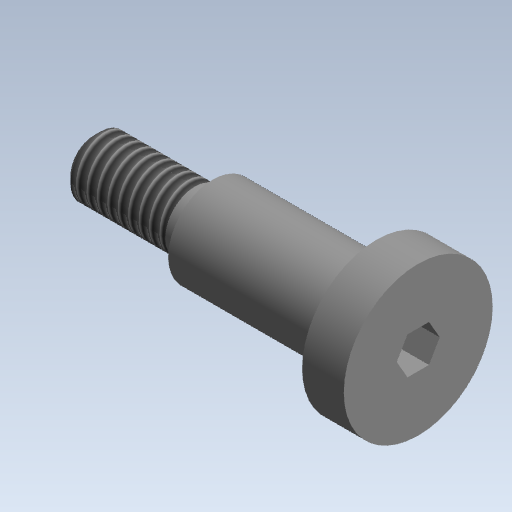
# Autodesk Inventor part: DBTS4-11-8
Saved by Autodesk Inventor 2020.4 (Build 244396000, 396)
## iProperties
Part Number: DBTS4-11-8
Material: 一般
Catalog Web Link: https://jp.misumi-ec.com/vona2/detail/110302679110/?HissuCode=DBTS4-11-8
Description: 既製品
Vendor: MISUMI
Document SubType Name: Modeling
Designer: partserver
Manufacturer: MISUMI
Mass: 0.615672 g
Surface Area: 5.71929 cm^2
Volume: 0.615672 cm^3
Density: 1 g/cm^3
Appearance: PSOLRGB-175-175-175
Category: PARTsolutions
Company: MISUMI
PSOL_IDENT_0: {$CADENAS_DATA\23d-libs\misumi\metric\27_screws_nuts\dbtb.prj},198 {VTYP=3D},{NB=DBTS4-11-8},{LINA=D
PSOL_IDENT_1: BTS4-11-8},{NN=DBTB, DBTM, DBTS},{DATE=03.06.2021 03:35:29},{GEOMDATE=06.03.2020 06:09:28},{VERSION=
PSOL_IDENT_2: },{LINEID=20},{WBVAR=MAT,ST,ALT1,L,F,ALT2,ALT3},{WBNUMERIC=L,F}  {NB=DBTS4-11-8},{LINA=DBTS4-11-8},{
PSOL_IDENT_3: KT=DUMMY},{PN=DBTS4-11-8},{TYPE=DBTS},{MAT=2},{ST=0},{ST0='0','-'},{M=4},{ALT1=},{L=11},{F=8},{FA=(3
PSOL_IDENT_4: :9/1)},{E=2.8},{D=6},{A=10},{B=2.5},{LL=1.2},{HH1=2.5},{P=0.7},{ALT2=},{GG=0.0},{FF=0.0},{LINC=[3:20
PSOL_IDENT_5: /1]},{ALT3=},{TOL=0/-0.2}
NB: DBTS4-11-8
NN: DBTB, DBTM, DBTS
NT: Stepped Bolts - Low Head Type
NBSYN: $PN.
LINA: DBTS4-11-8
CATALOG: Misumi
PN: DBTS4-11-8
MAT: 303 Stainless Steel
ST: -
M: 4
ALT1: w/o LTC (L Dimension Increment)
L: 11
F: 8
E: 2.8
D: 6
A: 10
B: 2.5
LL: 1.2
HH1: 2.5
ALT2: w/o PC (Relief on M)
ALT3: w/o DHC (Shaft Diameter Tolerance)
TOL: 0/-0.2
SUPPLIER: MISUMI
ARTICLENO: DBTS4-11-8
BOMINFO: DBTS4-11-8
CREATOR: CADENAS GmbH
Title: DBTS4-11-8
Author: Cadenas PARTsolutions
Comments: Stepped Bolts - Low Head Type
Autodesk Inventor part; units mm, degrees
ref_plane "YZ Plane" through (0, 0, 0) normal (1, 0, 0) x (0, 1, 0)
ref_plane "XZ Plane" through (0, 0, 0) normal (0, 1, 0) x (-1, 0, 0)
ref_plane "XY Plane" through (0, 0, 0) normal (0, 0, 1) x (1, 0, 0)
sketch "Sketch_1" plane through (0, 0, 0) normal (0, 0, 1) x (1, 0, 0)
  line L0 (11, 0) -> (-2.8, 0)
  line L1 (-2.8, 0) -> (-2.8, 5)
  line L2 (-2.8, 5) -> (0, 5)
  line L3 (0, 5) -> (0, 3)
  line L4 (0, 3) -> (11, 3)
  line L5 (11, 3) -> (11, 0)
  line L6 (11, 0) -> (-2.8, 0)
  constraints: 14 end point
revolve "Revolution1" add sketch "Sketch_1" angle 360 about axis through (11, 0, 0) along (1, 0, 0)
sketch "Sketch2" plane through (-2.8, 0, 0) normal (-1, 0, 0) x (0, 0, 1)
  point P0 (0, 0)
hole "Hole1" at (-2.8, 0, 0) direction (1, 0, 0) diameter 2.5 depth 2.5 tip angle 120
sketch "Sketch_3" plane through (-2.8, 0, 0) normal (1, 0, 0) x (0, 0, -1)
  line L0 (-1.25, -0.7217) -> (0, -1.4434)
  line L1 (0, -1.4434) -> (1.25, -0.7217)
  line L2 (1.25, -0.7217) -> (1.25, 0.7217)
  line L3 (1.25, 0.7217) -> (0, 1.4434)
  line L4 (0, 1.4434) -> (-1.25, 0.7217)
  line L5 (-1.25, 0.7217) -> (-1.25, -0.7217)
  constraints: 12 end point
extrude "Extrusion1" cut sketch "Sketch_3" along normal blind 2.5
sketch "Sketch_6" plane through (0, 0, 0) normal (0, 0, 1) x (1, 0, 0)
  line L0 (19, 0) -> (11, 0)
  line L1 (11, 0) -> (11, 2)
  line L2 (11, 2) -> (18.5705, 2)
  line L3 (18.5705, 2) -> (19, 1.5705)
  line L4 (19, 1.5705) -> (19, 0)
  line L5 (19, 0) -> (11, 0)
  constraints: 12 end point
revolve "Revolution2" add sketch "Sketch_6" angle 360 about axis through (19, 0, 0) along (1, 0, 0)
thread "Thread1" size "M4x0.7" class "6g" standard "ISO Metric profile" length 6.3705
body "Solid1"
